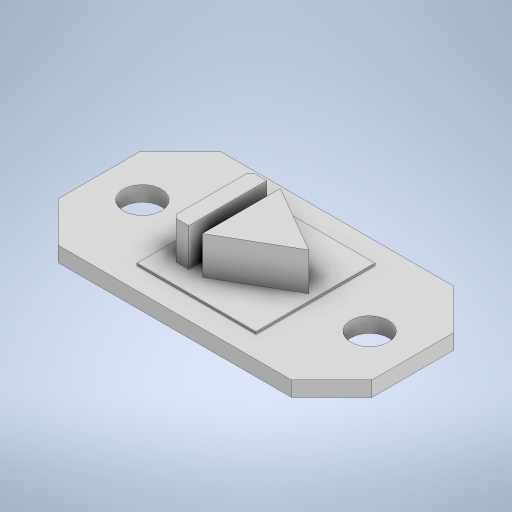
# Autodesk Inventor part: guzik_szablon
Saved by Autodesk Inventor 2024.3 (Build 283343000, 343)
## iProperties
Created: 2025-07-27
Part Number: guzik_szablon
Material: Ogólny
Document SubType Name: Modeling
Designer: User
Density: 1 g/cm^3
Appearance: Domyślna
Author: User
Autodesk Inventor part; units mm, degrees
ref_plane "YZ Plane" through (0, 0, 0) normal (1, 0, 0) x (0, 1, 0)
ref_plane "XZ Plane" through (0, 0, 0) normal (0, 1, 0) x (-1, 0, 0)
ref_plane "XY Plane" through (0, 0, 0) normal (0, 0, 1) x (1, 0, 0)
sketch "Szkic1" plane through (0, 0, 0) normal (0, 1, 0) x (-1, 0, 0)
  line L0 (-15, 8) -> (15, 8)
  line L1 (15, 8) -> (15, -8)
  line L2 (15, -8) -> (-15, -8)
  line L3 (-15, -8) -> (-15, 8)
  line L4 (-15, 8) -> (15, -8) construction
  line L5 (15, 8) -> (-15, -8) construction
  line L6 (-6, 6) -> (6, 6)
  line L7 (6, 6) -> (6, -6)
  line L8 (6, -6) -> (-6, -6)
  line L9 (-6, -6) -> (-6, 6)
  line L10 (-6, 6) -> (6, -6) construction
  line L11 (6, 6) -> (-6, -6) construction
  circle A0 centre (0, 0) radius 1.75
  dimension "d0" = 30
  dimension "d1" = 16
  dimension "d2" = 12
  dimension "d3" = 12
  dimension "d4" = 3.5
  constraints: 24 end point, 4 midpoint, 4 parallel, 2 horizontal, 2 perpendicular, 1 centre point, 1 coincident
  measures "d0" distance of L1.end L2.end
  measures "d1" distance of L0.end L1.end
  measures "d2" distance of L7.end L8.end
  measures "d3" distance of L6.end L7.end
  measures "d4" diameter of A0
extrude "Wyciągnięcie proste1" add sketch "Szkic1" along normal blind 1.4 contours L0 L1 L2 L3 | L6 L7 L8 L9 | A0
extrude "Wyciągnięcie proste2" add sketch "Szkic1" along normal blind 1.6 contours L6 L7 L8 L9 | A0
extrude "Wyciągnięcie proste3" cut sketch "Szkic1" along normal blind 1 contours A0
chamfer "Faza1" distance 4 angle 45 4 edges at (15, 0.7, 8) (15, 0.7, -8) (-15, 0.7, 8) (-15, 0.7, -8)
offset faces "Rozmiar1" outward -0.5 faces at (-3.6667, 0.4667, 8) (-12.3333, 0.4667, 6.6667) (12.3333, 0.4667, 6.6667) (15, 0.4667, 1.3333) (13.6667, 0.4667, -5.3333) (3.6667, 0.4667, -8) (-13.6667, 0.4667, -5.3333) (-15, 0.4667, -1.3333)
offset faces "Rozmiar2" outward -0.5 faces at (-2, 1.4667, 6) (6, 1.5333, -2) (-2, 1.5333, -6) (-6, 1.5333, 2)
sketch "Szkic2" plane through (0, 1.4, 0) normal (0, 1, 0) x (1, 0, 0)
  line L0 (-5.5, -5.5) -> (5.5, -5.5) projected
  line L1 (-5.5, 5.5) -> (5.5, 5.5) projected
  line L2 (-5.5, -5.5) -> (5.5, -5.5)
  line L3 (5.5, -5.5) -> (5.5, 5.5)
  line L4 (5.5, 5.5) -> (-5.5, 5.5)
  line L5 (-5.5, 5.5) -> (-5.5, -5.5)
  line L6 (0, 0) -> (-10.5, 0)
  line L7 (-10.5, 0) -> (10.5, 0)
  circle A0 centre (10.5, 0) radius 1.75
  circle A1 centre (-10.5, 0) radius 1.75
  dimension "d16" = 10.5
  dimension "d17" = 21
  dimension "d18" = 3.5
  dimension "d19" = 3.5
  constraints: 12 end point, 2 centre point, 2 coincident, 2 horizontal, 2 parallel, 1 perpendicular, 1 point on line
  measures "d16" distance of L6.start L6.end
  measures "d17" distance of L6.end L7.end
  measures "d18" diameter of A0
  measures "d19" diameter of A1
extrude "Wyciągnięcie proste4" cut sketch "Szkic2" against normal blind 10 contours A0 | A1
sketch "Szkic3" plane through (0, 1.6, 0) normal (0, 1, 0) x (1, 0, 0)
  line L0 (-5.2, 5.4) -> (5.4, 5.4)
  line L1 (5.4, 5.4) -> (5.4, -5.4)
  line L2 (-5.2, 5.4) -> (5.4, 5.4)
  line L3 (5.4, 5.4) -> (5.4, -5.4)
  line L4 (5.4, -5.4) -> (-5.2, -5.4)
  line L5 (-5.2, -5.4) -> (-5.2, 5.4)
  circle A0 centre (0.1, 0) radius 5.3
  line L6 (-5.2, 0) -> (5.4, 0)
  line L7 (-5.2, 0) -> (-3.85, 0)
  line L8 (-3.85, 0) -> (-3.85, 3.6)
  line L9 (-3.85, 3.6) -> (-2.35, 3.6)
  line L10 (-2.35, 3.6) -> (-2.35, 0)
  line L11 (-2.35, 0) -> (-1.35, 0)
  line L12 (-1.35, 0) -> (-1.35, 3.6)
  line L13 (-1.35, 3.6) -> (4.8854, 0)
  line L14 (-2.35, -3.6) -> (-2.35, 0)
  line L15 (-3.85, -3.6) -> (-2.35, -3.6)
  line L16 (-3.85, 0) -> (-3.85, -3.6)
  line L17 (-1.35, 0) -> (-1.35, -3.6)
  line L18 (-1.35, -3.6) -> (4.8854, 0)
  circle A1 centre (0.1, 0) radius 5.3
  circle A2 centre (0.1, 0) radius 7.65
  line L19 (-5.5, 5.5) -> (-5.5, -5.5) projected
  point P0 (0, 0)
  point P1 (-3.7897, 3.6)
  point P2 (-3.85, 3.5338)
  point P3 (-3.85, -3.5338)
  point P4 (-3.7897, -3.6)
  dimension "d22" = 1.35
  dimension "d23" = 3.6
  dimension "d24" = 90
  dimension "d25" = 1.5
  dimension "d26" = 90
  dimension "d27" = 1
  dimension "d28" = 3.6
  dimension "d29" = 60
  dimension "d30" = 15.3
  dimension "d33" = 1.65
  constraints: 38 end point, 6 point on line, 4 perpendicular, 3 centre point, 3 symmetric about line, 2 midpoint, 2 parallel, 2 point on circle, 1 coincident, 1 horizontal, 1 tangent, 1 other
  measures "d22" distance of L6.start L8.start
  measures "d23" distance of L8.start L8.end
  measures "d24" angle of L8 L7
  measures "d25" distance of L8.end L10.start
  measures "d26" angle of L8 L9
  measures "d27" distance of L10.end L11.end
  measures "d28" distance of L11.end L12.end
  measures "d29" angle of L12 L13
  measures "d30" diameter of A2
  measures "d33" distance between parallel lines of L8 L19
extrude "Wyciągnięcie proste5" add sketch "Szkic3" along normal blind 3.5 contours A0 L9 L10 L6 L8 | L16 L6 L14 L15 A0 | L18 L17 L6 | L6 L12 L13
move faces "Przesuń1" translate (-0.25, 0, 0) faces at (-2.35, 3.9333, 1.2) (-3.85, 2.7667, -1.1779)
move faces "Przesuń2" translate (0, -1.75, 0) faces at (-0.0229, 1, 0.3868)
